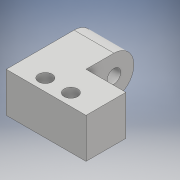
# Autodesk Inventor part: pixymount1
Saved by Autodesk Inventor 2017 (Build 210142000, 142)
## iProperties
Part Number: pixymount1
Material: 一般
Document SubType Name: Modeling
Designer: highs
Density: 1 g/cm^3
Appearance: 既定
Author: highs
## iProperties of the stored document pixymount1_3D プリント.ipt
Part Number: pixymount1_3D プリント
Material: 一般
Document SubType Name: Modeling
Designer: highs
Density: 1 g/cm^3
Appearance: 既定
Author: highs
Autodesk Inventor part; units mm, degrees
ref_plane "YZ Plane" through (0, 0, 0) normal (1, 0, 0) x (0, 1, 0)
ref_plane "XZ Plane" through (0, 0, 0) normal (0, 1, 0) x (-1, 0, 0)
ref_plane "XY Plane" through (0, 0, 0) normal (0, 0, 1) x (1, 0, 0)
sketch "スケッチ4" plane through (0, 0, 0) normal (0, 0, 1) x (1, 0, 0)
  line L0 (0, 0) -> (20, 0)
  line L1 (20, 0) -> (20, 10)
  line L2 (0, 22) -> (0, 0)
  line L3 (0, 22) -> (10, 22)
  line L4 (10, 22) -> (10, 10)
  line L5 (10, 10) -> (20, 10)
  line L6 (10, 0) -> (10, 7.8024) construction
  circle A0 centre (6.8, 3) radius 1.7
  circle A1 centre (13.2, 3) radius 1.7
  dimension "d19" = 20
  dimension "d20" = 22
  dimension "d21" = 12
  dimension "d22" = 10
  dimension "d23" = 6.4
  dimension "d24" = 3.4
  dimension "d25" = 3
  constraints: 14 end point, 3 horizontal, 2 centre point, 2 perpendicular, 1 midpoint, 1 parallel, 1 symmetric about line, 1 vertical, 1 other
  measures "d19" distance of L0.start L0.end
  measures "d20" distance of L2.start L0.start
  measures "d21" distance of L3.end L4.end
  measures "d22" distance of L2.start L3.end
  measures "d23" distance of A1.centre A0.centre
  measures "d24" diameter of A0
  measures "d25" distance from line of L0 A0.centre
extrude "押し出し4" add sketch "スケッチ4" along normal blind 10
sketch "スケッチ5" plane through (0, 0, 0) normal (-1, 0, 0) x (0, 0, 1)
  line L0 (0, 22) -> (10, 22) projected
  line L1 (5, 22) -> (5, 17) construction
  circle A0 centre (5, 17) radius 1.7
  point P0 (0, 0)
  dimension "d28" = 3.4
  dimension "d29" = 5
  constraints: 2 end point, 1 centre point, 1 coincident, 1 midpoint, 1 vertical
  measures "d28" diameter of A0
  measures "d29" distance from line of L0 A0.centre
extrude "押し出し5" cut sketch "スケッチ5" against normal blind 10
fillet "フィレット2" radius 5 2 edges at (5, 22, 0) (5, 22, 10)
